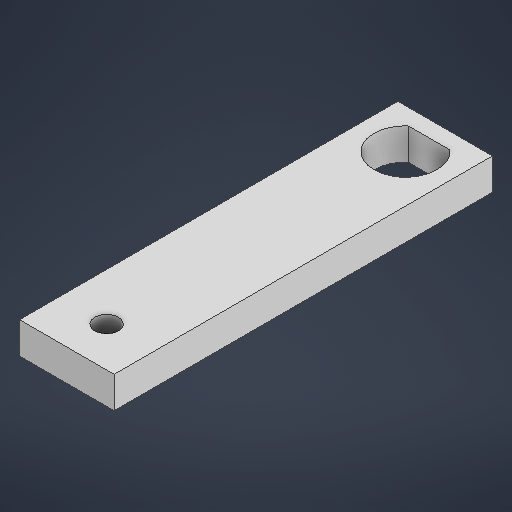
# Autodesk Inventor part: Virabrequim8
Saved by Autodesk Inventor 2026.2 (Build 302298000, 298)
## iProperties
Created: 2026-09-18
Part Number: Virabrequim8
Material: Genérico
Document SubType Name: Modeling
Designer: IFSP
Density: 1 g/cm^3
Appearance: Padrão
Author: IFSP
Autodesk Inventor part; units mm, degrees
ref_plane "YZ Plane" through (0, 0, 0) normal (1, 0, 0) x (0, 1, 0)
ref_plane "XZ Plane" through (0, 0, 0) normal (0, 1, 0) x (-1, 0, 0)
ref_plane "XY Plane" through (0, 0, 0) normal (0, 0, 1) x (1, 0, 0)
sketch "Esboço1" plane through (0, 0, 0) normal (0, 1, 0) x (-1, 0, 0)
  line L0 (9.525, 38.1) -> (-9.525, 38.1)
  line L1 (-9.525, 38.1) -> (-9.525, -38.1)
  line L2 (-9.525, -38.1) -> (9.525, -38.1)
  line L3 (9.525, -38.1) -> (9.525, 38.1)
  line L4 (9.525, 38.1) -> (-9.525, -38.1) construction
  line L5 (-9.525, 38.1) -> (9.525, -38.1) construction
  line L6 (0, -53.7953) -> (0, 49.8481)
  line L7 (-9.525, -38.1) -> (-9.525, -19.04) construction
  line L8 (-9.525, -19.04) -> (-9.525, 38.1) construction
  line L9 (0, -38.1) -> (0, -30.1) construction
  line L10 (0, 38.1) -> (0, 30.1) construction
  circle A0 centre (0, 30.1) radius 2.39
  arc A1 (4.205, -34.8582) -> (-4.205, -34.8582) centre (0, -30.1) ccw
  line L11 (-4.205, -34.8582) -> (4.205, -34.8582)
  point P0 (0, 0)
  dimension "d0" = 19.05
  dimension "d4" = 76.2
  dimension "d5" = 8
  dimension "d8" = 4.78
  dimension "d9" = 12.7
  constraints: 24 end point, 5 point on line, 4 midpoint, 2 centre point, 2 coincident, 2 parallel, 2 point on circle, 1 collinear, 1 horizontal, 1 perpendicular, 1 vertical
  measures "d0" distance of L2.end L1.end
  measures "d4" distance of L0.end L1.end
  measures "d5" distance of L9.start L9.end
  measures "d8" diameter of A0
  measures "d9" diameter of A1
extrude "Extrusão1" add sketch "Esboço1" along normal blind 6.35 contours L3 L2 L6 L11 A1 A0 L0 | L6 A0 A1 L11 L2 L1 L0
